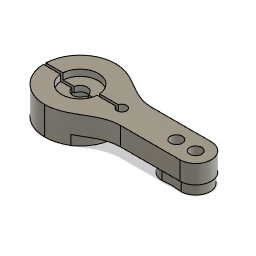
assembled new design (Autodesk Fusion 360 archive; units mm, degrees)
design "servo connector"
Autodesk Fusion 360 part; units mm, degrees
sketch "Sketch1" plane through (0, 0, 0) normal (0, 1, 0) x (1, 0, 0)
  circle A0 centre (0, 0) radius 7.35
  line L0 (0, -3.25) -> (24, -3.25)
  arc A1 (24, -3.25) -> (24, 3.25) centre (24, 0) ccw
  line L1 (24, 3.25) -> (0, 3.25)
  arc A2 (0, 3.25) -> (0, -3.25) centre (0, 0) ccw
  line L2 (0, 0) -> (24, 0) construction
  line L3 (-7.35, 0) -> (11.65, 0) construction
  line L4 (11.65, 0) -> (11.65, 3.25) construction
  circle A3 centre (24, 0) radius 1.25
  circle A4 centre (20, 0) radius 1.25
  spline S0 degree 5 poles (11.65, 3.25) (11.1355, 3.25) (10.1313, 3.3337) (8.6992, 3.7102) (6.9088, 4.6153) (4.7412, 5.9847) (2.9508, 6.8898) (1.5187, 7.2663) (0.5145, 7.35) (0, 7.35) knots 0 0 0 0 0 0 0.2 0.4 0.6 0.8 1 1 1 1 1 1
  line L5 (0, 7.35) -> (0, 0) construction
  spline S1 degree 5 poles (11.65, -3.25) (11.1355, -3.25) (10.1313, -3.3337) (8.6992, -3.7102) (6.9088, -4.6153) (4.7412, -5.9847) (2.9508, -6.8898) (1.5187, -7.2663) (0.5145, -7.35) (0, -7.35) knots 0 0 0 0 0 0 0.2 0.4 0.6 0.8 1 1 1 1 1 1
  line L6 (12.9681, 3.25) -> (10.3319, 3.25)
  line L7 (1.3181, 7.35) -> (-1.3181, 7.35)
  line L8 (12.9681, -3.25) -> (10.3319, -3.25)
  line L9 (1.3181, -7.35) -> (-1.3181, -7.35)
  circle A5 centre (0, 0) radius 1.5
  line L10 (-7.35, 0) -> (8.65, 0) construction
  circle A6 centre (8.65, 0) radius 1
  line L11 (8.65, 0.25) -> (-8, 0.25)
  arc A7 (-8, 0.25) -> (-8, -0.25) centre (-8, 0) ccw
  line L12 (-8, -0.25) -> (8.65, -0.25)
  arc A8 (8.65, -0.25) -> (8.65, 0.25) centre (8.65, 0) ccw
  line L13 (8.65, 0) -> (-8, 0) construction
  dimension "d1" = 14.7
  dimension "d4" = 24
  dimension "d5" = 6.5
  dimension "d6" = 19
  dimension "d7" = 4
  dimension "d8" = 2.5
  dimension "d9" = 2.5
  dimension "d10" = 3
  dimension "d11" = 16
  dimension "d12" = 2
  dimension "d15" = 0.5
  constraint coincident A0.centre A2.centre
  constraint tangent L0 A1
  constraint tangent A1 L1
  constraint parallel L0 L1
  constraint tangent L1 A2
  constraint tangent L0 A2
  constraint horizontal L2
  constraint coincident A0 L3.start
  constraint parallel L2 L3
  constraint coincident L1 L4.end
  constraint perpendicular L1 L4
  constraint concentric A1 A3
  constraint coincident L2 A4.centre
  constraint coincident A0 S0.end
  constraint perpendicular L3 L5
  constraint coincident S0.end L5.start
  constraint tangent A0 S0
  constraint midpoint L4.end L6
  constraint midpoint S0.end L7
  constraint symmetric L3 L4.end S1.start
  constraint symmetric L3 S0.end S1.end
  constraint symmetric L3 L6.start L8.start
  constraint symmetric L3 L6.end L8.end
  constraint symmetric L3 L7.start L9.start
  constraint symmetric L3 L7.end L9.end
  constraint perpendicular L4 L10
  constraint coincident L10.end A6.centre
  constraint tangent L11 A7
  constraint tangent A7 L12
  constraint parallel L11 L12
  constraint tangent L12 A8
  constraint tangent L11 A8
  constraint parallel L3 L13
  measures "d1" diameter of A0
  measures "d4" distance of A0.centre A1.centre
  measures "d5" diameter of A1
  measures "d6" distance of L3.start L3.end
  measures "d7" distance of A1.centre A4.centre
  measures "d8" diameter of A4
  measures "d9" diameter of A3
  measures "d10" diameter of A5
  measures "d11" distance of L3.start L10.end
  measures "d12" diameter of A6
  measures "d15" diameter of A7
extrude "Extrude1" add sketch "Sketch1" along normal blind 5.85 contours A0 L1 A2 A5 L11 | A0 L0 A1 L1 L6 L8 A6 L11 L12 | A0 L0 A2 A5 L12 | A0 L0 A2 L12 | A0 L1 A2 L11 | A0 L1 S0 L6 | A0 L0 S1 L8
sketch "Sketch2" plane through (0, 5.85, 0) normal (0, 1, 0) x (-1, 0, 0)
  circle A0 centre (-20, 0) radius 1.25
  circle A1 centre (-24, 0) radius 1.25
  line L0 (1.479, 0.25) -> (7.3457, 0.25)
  arc A2 (7.3457, 0.25) -> (0, 7.35) centre (0, 0) ccw
  spline S0 degree 5 poles (0, 7.35) (-0.5145, 7.35) (-1.5187, 7.2663) (-2.9508, 6.8898) (-4.7412, 5.9847) (-6.9088, 4.6153) (-8.6992, 3.7102) (-10.1313, 3.3337) (-11.1355, 3.25) (-11.65, 3.25) knots -1 -1 -1 -1 -1 -1 -0.8 -0.6 -0.4 -0.2 0 0 0 0 0 0
  line L1 (-11.65, 3.25) -> (-24, 3.25)
  arc A3 (-24, 3.25) -> (-24, -3.25) centre (-24, 0) ccw
  line L2 (-24, -3.25) -> (-11.65, -3.25)
  spline S1 degree 5 poles (-11.65, -3.25) (-11.1355, -3.25) (-10.1313, -3.3337) (-8.6992, -3.7102) (-6.9088, -4.6153) (-4.7412, -5.9847) (-2.9508, -6.8898) (-1.5187, -7.2663) (-0.5145, -7.35) (0, -7.35) knots 0 0 0 0 0 0 0.2 0.4 0.6 0.8 1 1 1 1 1 1
  arc A4 (0, -7.35) -> (7.3457, -0.25) centre (0, 0) ccw
  line L3 (7.3457, -0.25) -> (1.479, -0.25)
  arc A5 (-1.479, -0.25) -> (1.479, -0.25) centre (0, 0) ccw
  line L4 (-1.479, -0.25) -> (-7.6818, -0.25)
  arc A6 (-7.6818, 0.25) -> (-7.6818, -0.25) centre (-8.65, 0) ccw
  line L5 (-7.6818, 0.25) -> (-1.479, 0.25)
  arc A7 (1.479, 0.25) -> (-1.479, 0.25) centre (0, 0) ccw
  circle A8 centre (0, 0) radius 3.8
  dimension "d16" = 7.6
  constraint concentric A2 A8
  measures "d16" diameter of A8
extrude "Extrude2" cut sketch "Sketch2" against normal blind 1.3 contours L0 L5 A7 A8 | L3 A5 L4 A8
sketch "Sketch3" plane through (0, 0, 0) normal (0, -1, 0) x (1, 0, 0)
  circle A0 centre (20, 0) radius 1.25
  circle A1 centre (24, 0) radius 1.25
  line L0 (-7.3457, 0.25) -> (-1.479, 0.25)
  arc A2 (1.479, 0.25) -> (-1.479, 0.25) centre (0, 0) ccw
  line L1 (1.479, 0.25) -> (7.6818, 0.25)
  arc A3 (7.6818, -0.25) -> (7.6818, 0.25) centre (8.65, 0) ccw
  line L2 (7.6818, -0.25) -> (1.479, -0.25)
  arc A4 (-1.479, -0.25) -> (1.479, -0.25) centre (0, 0) ccw
  line L3 (-1.479, -0.25) -> (-7.3457, -0.25)
  arc A5 (-7.3457, -0.25) -> (0, -7.35) centre (0, 0) ccw
  spline S0 degree 5 poles (11.65, -3.25) (11.1355, -3.25) (10.1313, -3.3337) (8.6992, -3.7102) (6.9088, -4.6153) (4.7412, -5.9847) (2.9508, -6.8898) (1.5187, -7.2663) (0.5145, -7.35) (0, -7.35) knots 0 0 0 0 0 0 0.2 0.4 0.6 0.8 1 1 1 1 1 1
  line L4 (11.65, -3.25) -> (24, -3.25)
  arc A6 (24, -3.25) -> (24, 3.25) centre (24, 0) ccw
  line L5 (24, 3.25) -> (11.65, 3.25)
  spline S1 degree 5 poles (11.65, 3.25) (11.1355, 3.25) (10.1313, 3.3337) (8.6992, 3.7102) (6.9088, 4.6153) (4.7412, 5.9847) (2.9508, 6.8898) (1.5187, 7.2663) (0.5145, 7.35) (0, 7.35) knots 0 0 0 0 0 0 0.2 0.4 0.6 0.8 1 1 1 1 1 1
  arc A7 (0, 7.35) -> (-7.3457, 0.25) centre (0, 0) ccw
  circle A8 centre (0, 0) radius 2.95
  dimension "d19" = 5.9
  constraint concentric A2 A8
  measures "d19" diameter of A8
extrude "Extrude3" cut sketch "Sketch3" against normal blind 3.4 contours L0 A2 L1 A8 | L2 A4 L3 A8
sketch "Sketch4" plane through (0, 0, 0) normal (0, -1, 0) x (1, 0, 0)
  arc A0 (2.9394, 0.25) -> (-2.9394, 0.25) centre (0, 0) ccw
  line L0 (2.9394, 0.25) -> (7.6818, 0.25)
  arc A1 (7.6818, -0.25) -> (7.6818, 0.25) centre (8.65, 0) ccw
  line L1 (7.6818, -0.25) -> (2.9394, -0.25)
  arc A2 (-2.9394, -0.25) -> (2.9394, -0.25) centre (0, 0) ccw
  line L2 (-2.9394, -0.25) -> (-7.3457, -0.25)
  arc A3 (-7.3457, -0.25) -> (0, -7.35) centre (0, 0) ccw
  spline S0 degree 5 poles (11.65, -3.25) (11.1355, -3.25) (10.1313, -3.3337) (8.6992, -3.7102) (6.9088, -4.6153) (4.7412, -5.9847) (2.9508, -6.8898) (1.5187, -7.2663) (0.5145, -7.35) (0, -7.35) knots 0 0 0 0 0 0 0.2 0.4 0.6 0.8 1 1 1 1 1 1
  line L3 (11.65, -3.25) -> (24, -3.25)
  arc A4 (24, -3.25) -> (24, 3.25) centre (24, 0) ccw
  line L4 (24, 3.25) -> (11.65, 3.25)
  spline S1 degree 5 poles (11.65, 3.25) (11.1355, 3.25) (10.1313, 3.3337) (8.6992, 3.7102) (6.9088, 4.6153) (4.7412, 5.9847) (2.9508, 6.8898) (1.5187, 7.2663) (0.5145, 7.35) (0, 7.35) knots 0 0 0 0 0 0 0.2 0.4 0.6 0.8 1 1 1 1 1 1
  arc A5 (0, 7.35) -> (-7.3457, 0.25) centre (0, 0) ccw
  line L5 (-7.3457, 0.25) -> (-2.9394, 0.25)
  circle A6 centre (24, 0) radius 1.25
  circle A7 centre (20, 0) radius 1.25
  circle A8 centre (0, 0) radius 7.5
  circle A9 centre (20, 0) radius 1.25
  circle A10 centre (24, 0) radius 1.25
  circle A11 centre (20, 0) radius 3
  circle A12 centre (24, 0) radius 3
  line L6 (20, 0) -> (20, 3) construction
  line L7 (24, 0) -> (24, 3) construction
  line L8 (22, 2.2361) -> (22, 2.8361) construction
  spline S2 degree 5 poles (20, 3) (20.0835, 3) (20.2496, 2.9967) (20.496, 2.9819) (20.8196, 2.9457) (21.2171, 2.8903) (21.6098, 2.8451) (22, 2.8273) (22.3902, 2.8451) (22.7829, 2.8903) (23.1804, 2.9457) (23.504, 2.9819) (23.7504, 2.9967) (23.9165, 3) (24, 3) knots 0 0 0 0 0 0 0.1 0.2 0.3 0.4 0.5 0.6 0.7 0.8 0.9 1 1 1 1 1 1
  line L9 (20, 0) -> (24, 0) construction
  spline S3 degree 5 poles (20, -3) (20.0835, -3) (20.2496, -2.9967) (20.496, -2.9819) (20.8196, -2.9457) (21.2171, -2.8903) (21.6098, -2.8451) (22, -2.8273) (22.3902, -2.8451) (22.7829, -2.8903) (23.1804, -2.9457) (23.504, -2.9819) (23.7504, -2.9967) (23.9165, -3) (24, -3) knots 0 0 0 0 0 0 0.1 0.2 0.3 0.4 0.5 0.6 0.7 0.8 0.9 1 1 1 1 1 1
  line L10 (19.576, 3) -> (20.424, 3)
  line L11 (23.576, 3) -> (24.424, 3)
  line L12 (19.576, -3) -> (20.424, -3)
  line L13 (23.576, -3) -> (24.424, -3)
  point P0 (22, -2.8361)
  dimension "d22" = 1.75
  dimension "d23" = 1.75
  dimension "d24" = 0.6
  dimension "d27" = 15
  constraint concentric A0 A8
  constraint coincident A7.centre A9.centre
  constraint coincident A11 L6.end
  constraint vertical L6
  constraint coincident A4.centre A6.centre
  constraint coincident A12 L7.end
  constraint vertical L7
  constraint coincident A11 L8.start
  constraint coincident A12 L8.start
  constraint vertical L8
  constraint tangent A11 S2
  constraint tangent A12 S2
  constraint midpoint L6.end L10
  constraint midpoint L7.end L11
  constraint symmetric L6.end L9 S3.start
  constraint symmetric L7.end L9 S3.end
  constraint symmetric L8.end L9 P0
  constraint symmetric L9 L10.start L12.start
  constraint symmetric L9 L10.end L12.end
  constraint symmetric L9 L11.start L13.start
  constraint symmetric L9 L11.end L13.end
  measures "d24" distance of L8.start L8.end
  measures "d27" diameter of A8
extrude "Extrude4" cut sketch "Sketch4" against normal blind 2 contours L0 A1 L1 S0 L3 A4 L4 S1 A8

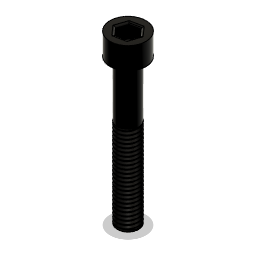
design "M6 45mmm"
Autodesk Fusion 360 part; units mm, degrees
sketch "Sketch1" plane through (0, 0, 0) normal (0, 1, 0) x (1, 0, 0)
  circle A0 centre (0, 0) radius 2.95
  dimension "d1" = 5.9
  constraint coincident A0.centre origin
  measures "d1" diameter of A0
extrude "Extrude1" add sketch "Sketch1" along normal blind 45.5
sketch "Sketch2" plane through (0, 45.5, 0) normal (0, 1, 0) x (-1, 0, 0)
  circle A0 centre (0, 0) radius 2.95
  circle A1 centre (0, 0) radius 4.875
  dimension "d4" = 9.75
  constraint coincident A0.centre A1.centre
  measures "d4" diameter of A1
extrude "Extrude2" add sketch "Sketch2" against normal blind 5.9
sketch "Sketch3" plane through (0, 45.5, 0) normal (0, 1, 0) x (-1, 0, 0)
  circle A0 centre (0, 0) radius 4.875
  line L0 (-2.8282, -0.5783) -> (-0.9133, -2.7385)
  line L1 (-0.9133, -2.7385) -> (1.9149, -2.1602)
  line L2 (1.9149, -2.1602) -> (2.8282, 0.5783)
  line L3 (2.8282, 0.5783) -> (0.9133, 2.7385)
  line L4 (0.9133, 2.7385) -> (-1.9149, 2.1602)
  line L5 (-1.9149, 2.1602) -> (-2.8282, -0.5783)
  dimension "d7" = 2.5
  constraint coincident A0.centre origin
  measures "d7" distance of A0.centre L5
extrude "Extrude3" cut sketch "Sketch3" against normal blind 3.85 contours L0 L1 L2 L3 L4 L5
fillet "Fillet1" radius 0.5 6 edges at (-2.3716, 45.5, -0.791) (-1.8708, 45.5, 1.6584) (0.5008, 45.5, 2.4493) (2.3716, 45.5, 0.791) (1.8708, 45.5, -1.6584) (-0.5008, 45.5, -2.4493)
fillet "Fillet1" radius 0.5 1 edges at (-2.7504, 0, 1.0668)
thread "Thread1" "ISO Metric profile 6.0 M6x1 6g" major diameter 5.884 minor diameter 4.7435 pitch 1 angle 60 modelled right hand crest width 0.1444 on face at (2.9463, 26.5667, 0.147) from (0, 0.5, 0) to (0, 24.5, 0) crest through (2.942, 0.25, 0)

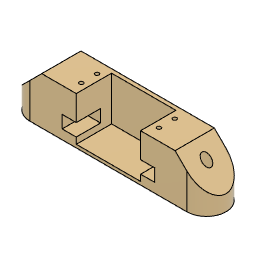
design "servo_base_fixture_new"
Autodesk Fusion 360 part; units mm, degrees
sketch "Sketch1" plane through (0, 0, 0) normal (0, 1, 0) x (1, 0, 0)
  line L0 (-62.5, 12.5) -> (62.5, 12.5)
  line L1 (62.5, 12.5) -> (62.5, -12.5)
  line L2 (62.5, -12.5) -> (-62.5, -12.5)
  line L3 (-62.5, -12.5) -> (-62.5, 12.5)
  line L4 (-62.5, 12.5) -> (62.5, -12.5) construction
  line L5 (62.5, 12.5) -> (-62.5, -12.5) construction
  dimension "d1" = 125
  dimension "d2" = 25
  constraint horizontal L0
  constraint perpendicular L0 L1
  constraint parallel L0 L2
  constraint parallel L1 L3
  constraint coincident L4 origin
  constraint coincident L5 origin
  measures "d1" distance of L1.end L2.end
  measures "d2" distance of L0.end L1.end
extrude "Extrude1" add sketch "Sketch1" along normal blind 30
sketch "Sketch3" plane through (0, 0, 12.5) normal (0, 0, 1) x (1, 0, 0)
  line L0 (-62.5, 0) -> (62.5, 0)
  line L1 (62.5, 0) -> (62.5, 30)
  line L2 (62.5, 30) -> (-62.5, 30)
  line L3 (-62.5, 30) -> (-62.5, 0)
  line L4 (-20.5, 30) -> (20.5, 30)
  line L5 (20.5, 30) -> (20.5, 2)
  line L6 (20.5, 2) -> (-20.5, 2)
  line L7 (-20.5, 2) -> (-20.5, 30)
  line L8 (-20.5, 14) -> (-29.5, 14)
  line L9 (-29.5, 14) -> (-29.5, 6)
  line L10 (-29.5, 6) -> (-20.5, 6)
  line L11 (-20.5, 6) -> (-20.5, 14)
  line L12 (0, 1.75) -> (0, 22.5)
  line L13 (0, 2) -> (0, 30) construction
  line L14 (20.5, 6) -> (20.5, 14)
  line L15 (29.5, 6) -> (20.5, 6)
  line L16 (29.5, 14) -> (29.5, 6)
  line L17 (20.5, 14) -> (29.5, 14)
  dimension "d5" = 28
  dimension "d8" = 12
  dimension "d9" = 8
  dimension "d10" = 9
  dimension "d11" = 41
  constraint horizontal L4
  constraint vertical L5
  constraint horizontal L6
  constraint vertical L7
  constraint coincident L2 L4.start
  constraint horizontal L8
  constraint vertical L9
  constraint horizontal L10
  constraint vertical L11
  constraint coincident L7 L8.start
  constraint midpoint L6 L13.start
  constraint midpoint L4 L13.end
  constraint symmetric L8.start L13 L14.end
  constraint symmetric L8.end L13 L16.start
  constraint symmetric L9.end L13 L15.start
  constraint symmetric L10.end L13 L14.start
  constraint symmetric L5 L7 L12
  measures "d5" distance of L4.start L6.end
  measures "d8" distance of L6 L8
  measures "d9" distance of L8.end L9.end
  measures "d10" distance of L8.start L8.end
  measures "d11" distance of L5 L7
extrude "Extrude2" cut sketch "Sketch3" against normal blind 22.5 contours L2 L4 L5 L6 L7 L11 L14
extrude "Extrude3" cut sketch "Sketch3" against normal blind 15.5 contours L2 L4 L5 L6 L7 L11 L14 | L7 L8 L9 L10 L11 | L5 L14 L15 L16 L17
chamfer "Chamfer1" distance 20 angle 45 2 edges at (-62.5, 30, 0) (62.5, 30, 0)
sketch "Sketch5" plane through (0, 30, 0) normal (0, 1, 0) x (-1, 0, 0)
  line L0 (-42.5, 12.5) -> (-42.5, -12.5)
  line L1 (-42.5, -12.5) -> (42.5, -12.5)
  line L2 (42.5, -12.5) -> (42.5, 12.5)
  line L3 (42.5, 12.5) -> (20.5, 12.5)
  line L4 (20.5, 12.5) -> (20.5, -10)
  line L5 (20.5, -10) -> (-20.5, -10)
  line L6 (-20.5, -10) -> (-20.5, 12.5)
  line L7 (-20.5, 12.5) -> (-42.5, 12.5)
  line L8 (24.75, -5) -> (-24.75, -5)
  line L9 (-24.75, -5) -> (-24.75, 5)
  line L10 (-24.75, 5) -> (24.75, 5)
  line L11 (24.75, 5) -> (24.75, -5)
  line L12 (24.75, -5) -> (-24.75, 5) construction
  line L13 (-24.75, -5) -> (24.75, 5) construction
  dimension "d23" = 49.5
  dimension "d24" = 10
  constraint horizontal L8
  constraint perpendicular L8 L9
  constraint parallel L8 L10
  constraint parallel L9 L11
  constraint coincident L12 origin
  constraint coincident L13 origin
  measures "d23" distance of L9.end L10.end
  measures "d24" distance of L8.end L9.end
hole "Hole1" at (-24.75, 30, -5) at (-24.75, 30, 5) at (24.75, 30, -5) at (24.75, 30, 5) direction (0, -1, 0) diameter 2.5 depth 12 tip angle 180
fillet "Fillet1" radius 12.5 4 edges at (62.5, 5, 12.5) (62.5, 5, -12.5) (-62.5, 5, 12.5) (-62.5, 5, -12.5)
sketch "Sketch6" plane through (0, 0, 0) normal (0, -1, 0) x (1, 0, 0)
  arc A0 (-50, 12.5) -> (-50, -12.5) centre (-50, 0) ccw
  line L0 (-50, -12.5) -> (50, -12.5)
  arc A1 (50, -12.5) -> (50, 12.5) centre (50, 0) ccw
  line L1 (50, 12.5) -> (-50, 12.5)
hole "Hole2" at (-50, 0, 0) at (50, 0, 0) direction (0, 1, 0) diameter 5.7 end through all
equation "d6 = -( 25 mm - 2.5 mm )"
equation "d13 = -( 25 mm - 2.5 mm - 7 mm )"

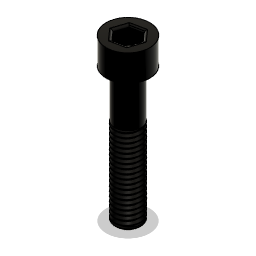
design "M6 30mm"
Autodesk Fusion 360 part; units mm, degrees
sketch "Sketch1" plane through (0, 0, 0) normal (0, 1, 0) x (1, 0, 0)
  circle A0 centre (0, 0) radius 2.95
  dimension "d1" = 5.9
  constraint coincident A0.centre origin
  measures "d1" diameter of A0
extrude "Extrude1" add sketch "Sketch1" along normal blind 36
sketch "Sketch2" plane through (0, 36, 0) normal (0, 1, 0) x (-1, 0, 0)
  circle A0 centre (0, 0) radius 2.95
  circle A1 centre (0, 0) radius 4.875
  dimension "d4" = 9.75
  constraint coincident A0.centre A1.centre
  measures "d4" diameter of A1
extrude "Extrude2" add sketch "Sketch2" against normal blind 5.9
sketch "Sketch3" plane through (0, 36, 0) normal (0, 1, 0) x (-1, 0, 0)
  circle A0 centre (0, 0) radius 4.875
  line L0 (-2.8282, -0.5783) -> (-0.9133, -2.7385)
  line L1 (-0.9133, -2.7385) -> (1.9149, -2.1602)
  line L2 (1.9149, -2.1602) -> (2.8282, 0.5783)
  line L3 (2.8282, 0.5783) -> (0.9133, 2.7385)
  line L4 (0.9133, 2.7385) -> (-1.9149, 2.1602)
  line L5 (-1.9149, 2.1602) -> (-2.8282, -0.5783)
  dimension "d7" = 2.5
  constraint coincident A0.centre origin
  measures "d7" distance of A0.centre L5
extrude "Extrude3" cut sketch "Sketch3" against normal blind 3.85 contours L0 L1 L2 L3 L4 L5
fillet "Fillet1" radius 0.5 6 edges at (-2.3716, 36, -0.791) (-1.8708, 36, 1.6584) (0.5008, 36, 2.4493) (2.3716, 36, 0.791) (1.8708, 36, -1.6584) (-0.5008, 36, -2.4493)
fillet "Fillet1" radius 0.5 1 edges at (-2.7504, 0, 1.0668)
thread "Thread1" "ISO Metric profile 6.0 M6x1 6g" major diameter 5.884 minor diameter 4.7435 pitch 1 angle 60 modelled right hand crest width 0.1444 on face at (2.9463, 20.2333, 0.147) from (0, 0.5, 0) to (0, 19.5, 0) crest through (2.942, 0.25, 0)

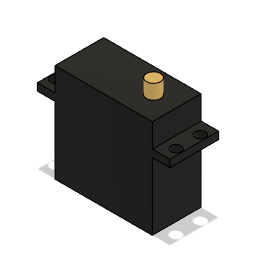
design "servo"
Autodesk Fusion 360 part; units mm, degrees
sketch "Sketch2" plane through (0, 0, 0) normal (0, 1, 0) x (1, 0, 0)
  line L0 (20, 10) -> (-20, 10)
  line L1 (-20, 10) -> (-20, -10)
  line L2 (-20, -10) -> (20, -10)
  line L3 (20, -10) -> (20, 10)
  line L4 (20, 10) -> (-20, -10) construction
  line L5 (-20, 10) -> (20, -10) construction
  dimension "d1" = 40
  dimension "d2" = 20
  constraint horizontal L0
  constraint perpendicular L0 L1
  constraint parallel L0 L2
  constraint parallel L1 L3
  constraint coincident L4 origin
  constraint coincident L5 origin
  measures "d1" distance of L1.end L2.end
  measures "d2" distance of L0.end L1.end
extrude "Extrude1" add sketch "Sketch2" along normal blind 40.4 makes body 1
ref_plane "WorkPlane1" through (0, 27.7, 0) normal (0, 1, 0) x (0, 0, 1)
sketch "Sketch3" plane through (0, 27.7, 0) normal (0, 1, 0) x (1, 0, 0)
  line L0 (-20, -10) -> (20, -10) construction
  line L1 (-20, 10) -> (-20, -10) construction
  line L2 (20, 10) -> (-20, 10) construction
  line L3 (20, -10) -> (20, 10) construction
  line L4 (27.25, -10) -> (-27.25, -10)
  line L5 (-27.25, -10) -> (-27.25, 10)
  line L6 (-27.25, 10) -> (27.25, 10)
  line L7 (27.25, 10) -> (27.25, -10)
  line L8 (27.25, -10) -> (-27.25, 10) construction
  line L9 (-27.25, -10) -> (27.25, 10) construction
  circle A0 centre (-24.75, 5) radius 2.125
  dimension "d6" = 54.5
  dimension "d7" = 20
  dimension "d10" = 4.25
  dimension "d11" = 5
  dimension "d12" = 24.75
  constraint horizontal L4
  constraint perpendicular L4 L5
  constraint parallel L4 L6
  constraint parallel L5 L7
  constraint coincident L8 origin
  constraint coincident L9 origin
  measures "d6" distance of L5.end L6.end
  measures "d7" distance of L4.end L5.end
  measures "d10" diameter of A0
  measures "d11" vertical distance of origin A0.centre
  measures "d12" horizontal distance of origin A0.centre
extrude "Extrude2" add sketch "Sketch3" along normal blind 3 contours L4 L5 L6 L7 | A0 bodies 1
extrude "Extrude3" cut sketch "Sketch3" along normal through all contours A0 bodies 1
pattern_linear "R-Pattern1" count 2 spacing 49.5 along (1, 0, 0) count 2 spacing 10 along (0, 0, 1) of "Extrude3"
sketch "Sketch4" plane through (0, 40.4, 0) normal (0, 1, 0) x (-1, 0, 0)
  line L0 (-20, 10) -> (-20, -10)
  line L1 (-20, -10) -> (20, -10)
  line L2 (20, -10) -> (20, 10)
  line L3 (20, 10) -> (-20, 10)
  circle A0 centre (-10.5, 0) radius 2.9
  dimension "d18" = 5.8
  dimension "d19" = 9.5
  measures "d18" diameter of A0
  measures "d19" distance of L0 A0.centre
extrude "Extrude4" add sketch "Sketch4" along normal blind 6 separate body contours A0 makes body 2
equation "d12 = ( 49.5 / 2 ) * 1 mm"

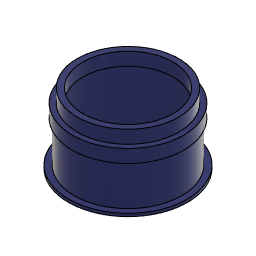
design "small end cap"
Autodesk Fusion 360 part; units mm, degrees
sketch "Sketch1" plane through (0, 0, 0) normal (0, 1, 0) x (1, 0, 0)
  circle A0 centre (0, 0) radius 18.5
  circle A1 centre (0, 0) radius 20.5
  circle A2 centre (0, 0) radius 17.5
  dimension "d1" = 37
  dimension "d2" = 2
  dimension "d3" = -1
  constraint coincident A0.centre A1.centre
  measures "d1" diameter of A0
extrude "Extrude1" add sketch "Sketch1" along normal blind 15 contours A0
extrude "Extrude2" add sketch "Sketch1" along normal blind 1 contours A1
sketch "Sketch2" plane through (0, 15, 0) normal (0, 1, 0) x (-1, 0, 0)
  circle A0 centre (0, 0) radius 17.5
  circle A1 centre (0, 0) radius 18.5
  circle A2 centre (0, 0) radius 17.5
  circle A3 centre (0, 0) radius 19.25
  dimension "d8" = 38.5
  constraint coincident A0.centre A1.centre
  measures "d8" diameter of A3
extrude "Extrude3" add sketch "Sketch2" along normal blind 4.5 contours A1 | A3
sketch "Sketch3" plane through (0, 19.5, 0) normal (0, 1, 0) x (-1, 0, 0)
  circle A0 centre (0, 0) radius 17.5
  circle A1 centre (0, 0) radius 19.25
  circle A2 centre (0, 0) radius 15.5
  circle A3 centre (0, 0) radius 17.5
  dimension "d11" = 31
  constraint concentric A0 A2
  measures "d11" diameter of A2
extrude "Extrude4" add sketch "Sketch3" along normal blind 4.5 contours A0 A3
sketch "Sketch4" plane through (0, 24, 0) normal (0, 1, 0) x (-1, 0, 0)
  circle A0 centre (0, 0) radius 15.5
  circle A1 centre (0, 0) radius 17.5
  circle A2 centre (0, 0) radius 12.5
  circle A3 centre (0, 0) radius 15.5
  dimension "d14" = 25
  constraint concentric A0 A2
  measures "d14" diameter of A2

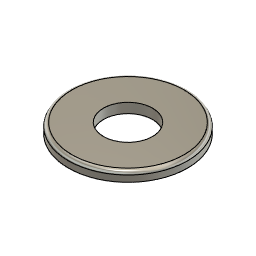
design "small washer"
Autodesk Fusion 360 part; units mm, degrees
sketch "Sketch1" plane through (0, 0, 0) normal (0, 1, 0) x (1, 0, 0)
  circle A0 centre (0, 0) radius 4.25
  circle A1 centre (0, 0) radius 1.75
  dimension "d1" = 8.5
  dimension "d2" = 3.5
  constraint coincident A0.centre A1.centre
  measures "d1" diameter of A0
  measures "d2" diameter of A1
extrude "Extrude1" add sketch "Sketch1" along normal blind 0.7
fillet "Fillet1" radius 0.25 1 edges at (-3.9624, 0.7, 1.5369)

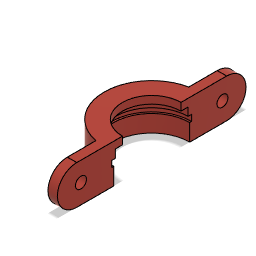
design "small end clamp TOP TEST fem"
Autodesk Fusion 360 part; units mm, degrees
sketch "Sketch1" plane through (0, 0, 0) normal (0, 1, 0) x (1, 0, 0)
  circle A0 centre (0, 0) radius 20.125
  circle A1 centre (0, 0) radius 25.125
  line L0 (5, 50) -> (-5, 50)
  line L1 (-5, 50) -> (-5, -50)
  line L2 (-5, -50) -> (5, -50)
  line L3 (5, -50) -> (5, 50)
  line L4 (5, 50) -> (-5, -50) construction
  line L5 (-5, 50) -> (5, -50) construction
  dimension "d1" = 40.25
  dimension "d2" = 5
  dimension "d3" = 10
  dimension "d4" = 100
  constraint coincident A0.centre A1.centre
  constraint horizontal L0
  constraint perpendicular L0 L1
  constraint parallel L0 L2
  constraint parallel L1 L3
  constraint coincident L4 A0.centre
  constraint coincident L5 A0.centre
  measures "d1" diameter of A0
  measures "d3" distance of L1.end L2.end
  measures "d4" distance of L0.end L1.end
extrude "Extrude1" add sketch "Sketch1" along normal blind 9 contours A0 A1 L3 | A0 A1 L1 L3 | A0 A1 L1 L3 | A0 A1 L1 | A1 L0 L1 L3 | A1 L1 L2 L3 makes body 1
sketch "Sketch2" plane through (0, 9, 0) normal (0, 1, 0) x (-1, 0, 0)
  circle A0 centre (0, 0) radius 20.125
  line L0 (-5, 50) -> (-5, 24.6225)
  arc A1 (-5, 24.6225) -> (-5, -24.6225) centre (0, 0) ccw
  line L1 (-5, -24.6225) -> (-5, -50)
  line L2 (-5, -50) -> (5, -50)
  line L3 (5, -50) -> (5, -24.6225)
  arc A2 (5, -24.6225) -> (5, 24.6225) centre (0, 0) ccw
  line L4 (5, 24.6225) -> (5, 50)
  line L5 (5, 50) -> (-5, 50)
  circle A3 centre (0, 0) radius 21.15
  dimension "d7" = 42.3
  constraint concentric A0 A3
  measures "d7" diameter of A3
extrude "Extrude2" add sketch "Sketch2" along normal blind 3.25 contours L0 A1 L1 L2 L3 A2 L4 L5 bodies 1
sketch "Sketch3" plane through (0, 12.25, 0) normal (0, 1, 0) x (-1, 0, 0)
  circle A0 centre (0, 0) radius 21.15
  line L0 (5, 50) -> (-5, 50)
  line L1 (-5, 50) -> (-5, 24.6225)
  arc A1 (-5, 24.6225) -> (-5, -24.6225) centre (0, 0) ccw
  line L2 (-5, -24.6225) -> (-5, -50)
  line L3 (-5, -50) -> (5, -50)
  line L4 (5, -50) -> (5, -24.6225)
  arc A2 (5, -24.6225) -> (5, 24.6225) centre (0, 0) ccw
  line L5 (5, 24.6225) -> (5, 50)
  circle A3 centre (0, 0) radius 19.25
  dimension "d10" = 38.5
  constraint coincident A0.centre A1.centre
  measures "d10" diameter of A3
extrude "Extrude3" add sketch "Sketch3" along normal blind 4.3 contours A0 | L0 L1 A1 L2 L3 L4 A2 L5 bodies 1
sketch "Sketch4" plane through (0, 16.55, 0) normal (0, 1, 0) x (-1, 0, 0)
  circle A0 centre (0, 0) radius 19.25
  line L0 (5, 24.6225) -> (5, 50)
  line L1 (5, 50) -> (-5, 50)
  line L2 (-5, 50) -> (-5, 24.6225)
  arc A1 (-5, 24.6225) -> (-5, -24.6225) centre (0, 0) ccw
  line L3 (-5, -24.6225) -> (-5, -50)
  line L4 (-5, -50) -> (5, -50)
  line L5 (5, -50) -> (5, -24.6225)
  arc A2 (5, -24.6225) -> (5, 24.6225) centre (0, 0) ccw
  circle A3 centre (0, 0) radius 15.5
  dimension "d13" = 31
  constraint coincident A0.centre A1.centre
  measures "d13" diameter of A3
extrude "Extrude4" add sketch "Sketch4" along normal blind 4 contours A0 | L0 L1 L2 A1 L3 L4 L5 A2 bodies 1
fillet "Fillet1" [suppressed]
sketch "Sketch5" plane through (5, 0, 0) normal (1, 0, 0) x (0, 0, -1)
  line L0 (-50, 0) -> (-24.6225, 0)
  line L1 (-24.6225, 0) -> (-24.6225, 20.55)
  line L2 (-24.6225, 20.55) -> (-50, 20.55)
  line L3 (-50, 20.55) -> (-50, 0)
  circle A0 centre (-37.5, 10.275) radius 2.95
  dimension "d17" = 5.9
  dimension "d20" = 37.5
  dimension "d21" = 10.275
  measures "d17" diameter of A0
  measures "d20" horizontal distance of origin A0.centre
  measures "d21" distance of L2 A0.centre
extrude "Extrude5" cut sketch "Sketch5" against normal through all contours A0 bodies 1
mirror "Mirror1" about plane through (0, 0, 0) normal (0, 0, 1) of 1 faces at (1.6667, 9.9813, 34.5647) on bodies 1
split "Split1" by plane through (0, 0, 0) normal (1, 0, 0) bodies 1 makes body 2 at (6.1778, 6.85, 24.3537)
sketch "Sketch6" plane through (0, 0, 0) normal (0, 1, 0) x (1, 0, 0)
fillet "Fillet2" radius 10.275 4 edges at (-2.5, 20.55, 50) (-2.5, 0, 50) (-2.5, 20.55, -50) (-2.5, 0, -50) on bodies 1
hidden bodies 2
equation "d20 = ( 75 / 2 ) * 1 mm"
equation "d21 = ( 20.55 / 2 ) * 1 mm"
equation "d22 = 20.55 mm / 2"
named bodies: "top", "bottom"

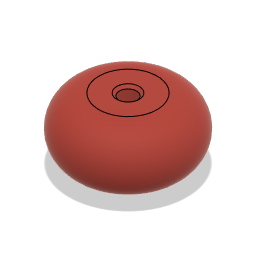
design "roller_bl"
Autodesk Fusion 360 part; units mm, degrees
sketch "Sketch1" plane through (0, 0, 0) normal (0, 1, 0) x (1, 0, 0)
  circle A0 centre (0, 0) radius 22.5
  circle A1 centre (0, 0) radius 3.25
  dimension "d1" = 45
  dimension "d5" = 6.5
  constraint coincident A0.centre A1.centre
  measures "d1" diameter of A0
  measures "d5" diameter of A1
extrude "Extrude1" add sketch "Sketch1" along normal blind 23
fillet "Fillet1" radius 11.5 2 edges at (-20.9774, 23, 8.1363) (-20.9774, 0, 8.1363)
chamfer "Chamfer1" distance 1 angle 45 2 edges at (-3.0301, 23, -1.1753) (-3.0301, 0, -1.1753)
equation "d4 = ( 23 / 2 ) * 1 mm"
